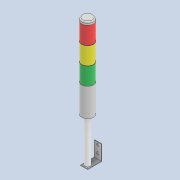
# Autodesk Inventor part: Signal Tower
Saved by Autodesk Inventor 2022 (Build 260153000, 153)
## iProperties
Created: 2021-10-30
Part Number: Signal Tower
Material: Generic
Document SubType Name: Modeling
Designer: Coy
Density: 1 g/cm^3
Appearance: Default
Author: Coy
Autodesk Inventor part; units mm, degrees
ref_plane "YZ Plane" through (0, 0, 0) normal (1, 0, 0) x (0, 1, 0)
ref_plane "XZ Plane" through (0, 0, 0) normal (0, 1, 0) x (-1, 0, 0)
ref_plane "XY Plane" through (0, 0, 0) normal (0, 0, 1) x (1, 0, 0)
sketch "Sketch1" plane through (0, 0, 0) normal (0, 1, 0) x (-1, 0, 0)
  line L0 (0, 0) -> (24, 0)
  line L1 (24, 0) -> (24, -48)
  line L2 (24, -48) -> (0, -48)
  line L3 (0, -48) -> (0, 0)
  line L4 (12, 0) -> (12, -48) construction
  circle A0 centre (12, -12) radius 9 construction
  dimension "d0" = 18
  dimension "d1" = 3
  dimension "d2" = 3
  dimension "d3" = 48
  constraints: 10 end point, 2 midpoint, 2 parallel, 1 centre point, 1 horizontal, 1 perpendicular, 1 point on line
  measures "d0" diameter of A0
  measures "d1" distance edge to line of A0 L0
  measures "d2" distance edge to line of A0 L1
  measures "d3" distance of L0.end L1.end
extrude "Extrusion1" add sketch "Sketch1" along normal blind 2
sketch "Sketch2" plane through (0, 2, 0) normal (0, 1, 0) x (1, 0, 0)
  line L0 (-24, 48) -> (-24, 0) projected
  line L1 (0, 0) -> (0, 48) projected
  line L2 (-24, 48) -> (0, 48)
  line L3 (0, 48) -> (0, 46)
  line L4 (0, 46) -> (-24, 46)
  line L5 (-24, 46) -> (-24, 48)
  dimension "d6" = 2
  constraints: 8 end point, 2 parallel, 1 horizontal, 1 perpendicular, 1 point on line
  measures "d6" distance of L2.end L3.end
extrude "Extrusion2" add sketch "Sketch2" along normal blind 50
sketch "Sketch3" plane through (-24, 2, -46) normal (0, 0, 1) x (1, 0, 0)
  line L0 (24, 50) -> (0, 50) construction
  line L1 (12, 50) -> (12, 0) construction
  line L2 (0, 0) -> (24, 0) construction
  line L3 (12, 47) -> (12, 37) construction
  line L4 (9, 44) -> (9, 40)
  line L5 (15, 40) -> (15, 44)
  arc A0 (15, 44) -> (9, 44) centre (12, 44) ccw
  arc A1 (9, 40) -> (15, 40) centre (12, 40) ccw
  line L6 (12, 22) -> (12, 12) construction
  line L7 (9, 19) -> (9, 15)
  line L8 (15, 15) -> (15, 19)
  arc A2 (15, 19) -> (9, 19) centre (12, 19) ccw
  arc A3 (9, 15) -> (15, 15) centre (12, 15) ccw
  point P0 (24, -2)
  point P1 (12, 42)
  point P2 (12, 17)
  dimension "d9" = 6
  dimension "d10" = 10
  dimension "d11" = 3
  dimension "d12" = 10
  dimension "d13" = 6
  dimension "d14" = 15
  constraints: 18 end point, 12 point on circle, 8 point on line, 8 tangent, 4 centre point, 4 midpoint, 2 parallel
  measures "d9" diameter of A1
  measures "d10" distance of L3.start L3.end
  measures "d11" distance from line of L0 L3.start
  measures "d12" distance of L6.start L6.end
  measures "d13" diameter of A3
  measures "d14" distance of L3.end L6.start
extrude "Extrusion3" cut sketch "Sketch3" against normal up to next
sketch "Sketch4" plane through (0, 2, 0) normal (0, 1, 0) x (1, 0, 0)
  line L0 (-24, 0) -> (0, 0) construction
  line L1 (-12, 0) -> (-12, 46) construction
  line L2 (-9, 46) -> (-15, 46) construction
  circle A0 centre (-12, 11.5) radius 8.5
  dimension "d17" = 17
  dimension "d18" = 3
  constraints: 2 end point, 2 midpoint, 1 centre point, 1 point on line
  measures "d17" diameter of A0
  measures "d18" distance edge to line of A0 L0
extrude "Extrusion4" add sketch "Sketch4" along normal blind 150
sketch "Sketch5" plane through (-12, 152, -11.5) normal (0, 1, 0) x (1, 0, 0)
  circle A0 centre (0, 0) radius 8.5 projected
  circle A1 centre (0, 0) radius 20
  point P0 (12, -11.5)
  dimension "d21" = 40
  constraints: 1 centre point, 1 coincident
  measures "d21" diameter of A1
extrude "Extrusion5" add sketch "Sketch5" along normal blind 95 contours A0 | A1
sketch "Sketch6" plane through (-12, 247, -11.5) normal (0, 1, 0) x (1, 0, 0)
  circle A0 centre (0, 0) radius 20 projected
  circle A1 centre (0, 0) radius 19.9
  point P0 (12, -11.5)
  dimension "d24" = 0.1
  constraints: 1 centre point
  measures "d24" radial gap between concentric circles of A0 A1
sketch "Sketch6 outline for Extrusion6" plane through (-12, 247, -11.5) normal (0, 1, 0) x (1, 0, 0)
  circle A0 centre (0, 0) radius 19.9
extrude "Extrusion6" add sketch "Sketch6 outline for Extrusion6" along normal blind 59
sketch "Sketch7" plane through (-12, 306, -11.5) normal (0, 1, 0) x (1, 0, 0)
  circle A0 centre (0, 0) radius 19.9 projected
  circle A1 centre (0, 0) radius 20
  point P0 (12, -11.5)
  dimension "d27" = 0.1
  constraints: 1 centre point
  measures "d27" radial gap between concentric circles of A0 A1
extrude "Extrusion7" add sketch "Sketch7" along normal blind 1 contours A0 | A1
sketch "Sketch8" plane through (-12, 307, -11.5) normal (0, 1, 0) x (1, 0, 0)
  circle A0 centre (0, 0) radius 19.9 projected
  point P0 (12, -11.5)
extrude "Extrusion8" add sketch "Sketch8" along normal blind 59
sketch "Sketch9" plane through (-12, 366, -11.5) normal (0, 1, 0) x (1, 0, 0)
  circle A0 centre (0, 0) radius 19.9 projected
  circle A1 centre (0, 0) radius 20 projected
  point P0 (12, -11.5)
extrude "Extrusion9" add sketch "Sketch9" along normal blind 1 contours A0 | A1
sketch "Sketch10" plane through (-12, 367, -11.5) normal (0, 1, 0) x (1, 0, 0)
  circle A0 centre (0, 0) radius 19.9 projected
  point P0 (12, -11.5)
extrude "Extrusion10" add sketch "Sketch10" along normal blind 59
sketch "Sketch11" plane through (-12, 426, -11.5) normal (0, 1, 0) x (1, 0, 0)
  circle A0 centre (0, 0) radius 20 projected
  point P0 (12, -11.5)
extrude "Extrusion11" add sketch "Sketch11" along normal blind 10
fillet "Fillet1" radius 4 1 edges at (-32, 436, -11.5)
fillet "Fillet2" radius 5 1 edges at (-20.5, 152, -11.5)
equation "\"d2\" = d1"
body "Solid1"
